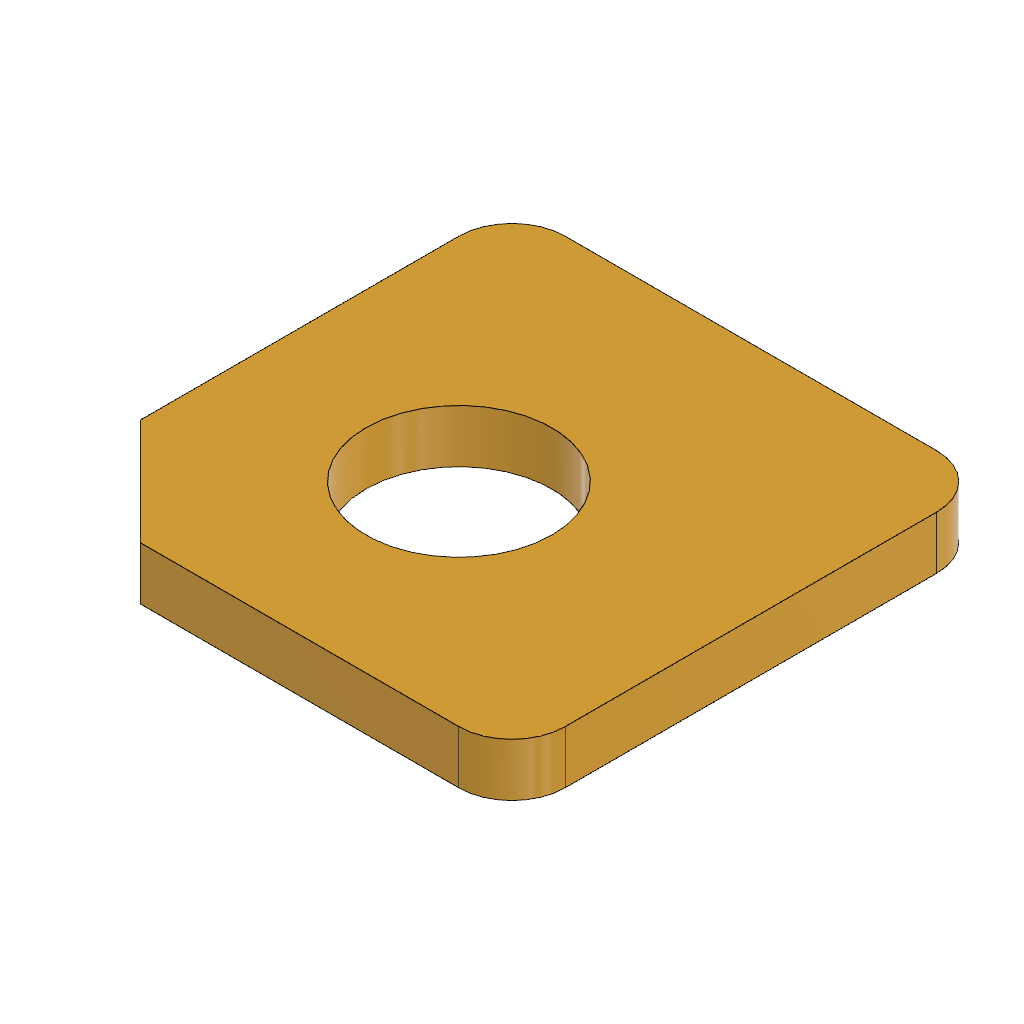
BasePlate (Autodesk Fusion 360 design; units mm, degrees)
part number: 2026-07-26-22-50-56-387
Autodesk Fusion 360 part; units mm, degrees
sketch "Sketch1" plane through (0, 0, 0) normal (0, 0, 1) x (1, 0, 0)
  line L0 (9.6355, -4.918) -> (79.6355, -4.918)
  line L1 (89.6355, -14.918) -> (89.6355, -84.918)
  line L2 (79.6355, -94.918) -> (-0.3645, -94.918)
  line L3 (-0.3645, -94.918) -> (-0.3645, -14.918)
  line L4 (-0.3645, -74.918) -> (19.6355, -94.918)
  circle A0 centre (39.6355, -54.918) radius 17.5
  arc A1 (9.6355, -4.918) -> (-0.3645, -14.918) centre (9.6355, -14.918) ccw
  arc A2 (89.6355, -14.918) -> (79.6355, -4.918) centre (79.6355, -14.918) ccw
  arc A3 (79.6355, -94.918) -> (89.6355, -84.918) centre (79.6355, -84.918) ccw
  point P0 (-0.3645, -4.918)
  point P1 (89.6355, -4.918)
  dimension "d1" = 90
  dimension "d2" = 90
  dimension "d3" = 20
  dimension "d4" = 20
  dimension "d5" = 35
  dimension "d6" = 40
  dimension "d7" = 40
  dimension "d8" = 10
  dimension "d9" = 10
  dimension "d10" = 10
  constraint horizontal L0
  constraint vertical L1
  constraint horizontal L2
  constraint vertical L3
  constraint coincident L3 L4.start
  constraint coincident L2 L4.end
  constraint coincident P0 L3
  constraint coincident P0 L0
  constraint tangent L3 A1
  constraint tangent L0 A1
  constraint coincident P1 L0
  constraint coincident P1 L1
  constraint tangent L0 A2
  constraint tangent L1 A2
  constraint tangent L1 A3
  constraint tangent L2 A3
  measures "d1" distance of P0 P1
  measures "d2" distance of P0 L2.end
  measures "d3" vertical distance of L4.start L4.end
  measures "d4" distance of L3 L4.end
  measures "d5" diameter of A0
  measures "d6" distance of L3 A0.centre
  measures "d7" distance of L2 A0.centre
  measures "d8" radius of A1
  measures "d9" radius of A2
  measures "d10" radius of A3
extrude "Extrude1" add sketch "Sketch1" along normal blind 10 contours L0 L1 L2 L3 L4 A1 A2 A3
